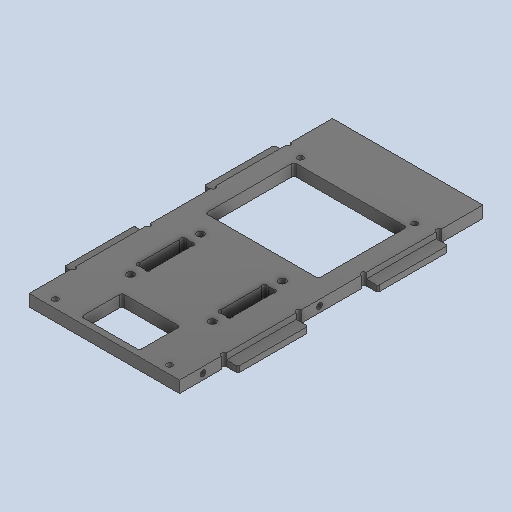
# Autodesk Inventor part: Cockpit_upper_bottom_frame
Saved by Autodesk Inventor 2022.4 (Build 264492000, 492)
## iProperties
Created: 2021-04-13
Part Number: Cockpit_upper_bottom_frame
Material: アセタール樹脂、黒
Document SubType Name: Modeling
Designer: Masato Kubotera
Density: 1.425 g/cm^3
Appearance: 滑らか - 黒
Mass: 43.5821 g
Surface Area: 172.155 cm^2
Volume: 30.5839 cm^3
Description: POM T5
d0: 64.500 mm
d1: 130.000 mm
d2: 20.000 mm
d3: 30.000 mm
d4: 30.000 mm
d5: 30.000 mm
d6: 1.050 mm
d7: 1.050 mm
d8: 1.050 mm
d9: 1.050 mm
d10: 5.000 mm
d23: 15.000 mm
d24: 5.000 mm
d25: 20.000 mm
d28: 3.100 mm
d66: 2.500 mm
d67: 0.00 deg
d68: 5.000 mm
d69: 0.00 deg
d72: 47.500 mm
d101: 1.000 mm
d103: 12.250 mm
d109: 71.250 mm
Author: Masato Kubotera
Title: Cockpit_horizontal_frame_02
Autodesk Inventor part; units mm, degrees
ref_plane "YZ Plane" through (0, 0, 0) normal (1, 0, 0) x (0, 1, 0)
ref_plane "XZ Plane" through (0, 0, 0) normal (0, 1, 0) x (-1, 0, 0)
ref_plane "XY Plane" through (0, 0, 0) normal (0, 0, 1) x (1, 0, 0)
sketch "スケッチ1" plane through (0, 0, 0) normal (0, 0, 1) x (1, 0, 0)
  line L0 (-32.25, 65) -> (32.25, 65)
  line L1 (32.25, 65) -> (32.25, 47.1)
  line L2 (-32.25, -65) -> (-32.25, -47.1)
  line L3 (-32.25, 65) -> (32.25, -65) construction
  line L4 (32.25, 65) -> (-32.25, -65) construction
  line L5 (-32.25, 45) -> (-37.25, 45)
  line L6 (-37.25, 15) -> (-32.25, 15)
  line L7 (-37.25, 15) -> (-37.25, 45)
  line L8 (-32.25, -15) -> (-37.25, -15)
  line L9 (-37.25, -15) -> (-37.25, -45)
  line L10 (-37.25, -45) -> (-32.25, -45)
  arc A0 (-32.25, 45) -> (-32.25, 47.1) centre (-32.25, 46.05) ccw
  arc A1 (-32.25, 12.9) -> (-32.25, 15) centre (-32.25, 13.95) ccw
  arc A2 (-32.25, -15) -> (-32.25, -12.9) centre (-32.25, -13.95) ccw
  arc A3 (-32.25, -47.1) -> (-32.25, -45) centre (-32.25, -46.05) ccw
  line L11 (-32.25, 47.1) -> (-32.25, 65)
  line L12 (-32.25, 12.9) -> (-32.25, 15) construction
  line L13 (-32.25, -12.9) -> (-32.25, 12.9)
  line L14 (-32.25, -47.1) -> (-32.25, -45) construction
  line L15 (0, 65) -> (0, -65) construction
  arc A4 (32.25, -45) -> (32.25, -47.1) centre (32.25, -46.05) ccw
  line L16 (37.25, -45) -> (32.25, -45)
  line L17 (37.25, -15) -> (37.25, -45)
  line L18 (32.25, -15) -> (37.25, -15)
  arc A5 (32.25, -12.9) -> (32.25, -15) centre (32.25, -13.95) ccw
  arc A6 (32.25, 15) -> (32.25, 12.9) centre (32.25, 13.95) ccw
  line L19 (37.25, 15) -> (37.25, 45)
  line L20 (37.25, 15) -> (32.25, 15)
  line L21 (32.25, 45) -> (37.25, 45)
  arc A7 (32.25, 47.1) -> (32.25, 45) centre (32.25, 46.05) ccw
  line L22 (32.25, 47.1) -> (32.25, 45) construction
  line L23 (32.25, 12.9) -> (32.25, -12.9)
  line L24 (32.25, -47.1) -> (32.25, -65)
  line L25 (32.25, -12.9) -> (32.25, -15) construction
  line L26 (-32.25, -15) -> (-32.25, -12.9) construction
  line L27 (-32.25, -45) -> (-32.25, -15)
  line L28 (32.25, -15) -> (32.25, -45)
  line L29 (32.25, -45) -> (32.25, -47.1) construction
  line L30 (-20, -11.25) -> (-15, -11.25) construction
  line L31 (-15, -11.25) -> (-15, -31.25) construction
  line L32 (-15, -31.25) -> (-20, -31.25) construction
  line L33 (-20, -31.25) -> (-20, -11.25) construction
  line L34 (-20, -11.25) -> (-15, -31.25) construction
  line L35 (-15, -11.25) -> (-20, -31.25) construction
  line L36 (-20, 2.5) -> (-15, 2.5) construction
  line L37 (-15, 2.5) -> (-15, -45) construction
  line L38 (-15, -45) -> (-20, -45) construction
  line L39 (-20, -45) -> (-20, 2.5) construction
  line L40 (-20, 2.5) -> (-15, -45) construction
  line L41 (-15, 2.5) -> (-20, -45) construction
  circle A8 centre (-17.5, -36.25) radius 1.55
  line L42 (-20, -21.25) -> (-15, -21.25) construction
  line L43 (-17.5, 2.5) -> (-17.5, -45) construction
  circle A9 centre (-17.5, -6.25) radius 1.55
  circle A10 centre (17.5, -36.25) radius 1.55
  circle A11 centre (17.5, -6.25) radius 1.55
  line L44 (32.25, -65) -> (16.75, -65)
  line L45 (-12.5, -62.5) -> (-12.5, -45)
  line L46 (-12.5, -45) -> (0, -45)
  line L47 (12.5, -62.5) -> (12.5, -45)
  line L48 (12.5, -45) -> (0, -45)
  line L49 (-16.75, -65) -> (-32.25, -65)
  line L50 (16.75, -65) -> (-16.75, -65)
  line L51 (-32.25, 45) -> (-32.25, 47.1) construction
  line L52 (-32.25, 15) -> (-32.25, 45)
  line L53 (32.25, 15) -> (32.25, 12.9) construction
  line L54 (32.25, 45) -> (32.25, 15)
  circle A12 centre (-24.5, 43.5) radius 1.25
  line L55 (-32.25, 0) -> (32.25, 0) construction
  line L56 (-32.25, 46.5) -> (32.25, 46.5) construction
  circle A13 centre (-24.5, -61.5) radius 1.25
  circle A14 centre (24.5, 43.5) radius 1.25
  circle A15 centre (24.5, -61.5) radius 1.25
  circle A16 centre (-17.5, -36.25) radius 3 construction
  line L57 (-12.5, -62.5) -> (12.5, -62.5)
  line L58 (-24.25, 40.5) -> (24.25, 40.5)
  line L59 (24.25, 2.5) -> (-24.25, 2.5)
  line L60 (-24.25, 2.5) -> (-24.25, 40.5)
  line L61 (24.25, 2.5) -> (24.25, 40.5)
  line L62 (-20.05, -29.8151) -> (-18.5651, -31.3) construction
  line L63 (-19.3075, -30.5575) -> (-20.05, -31.3) construction
  arc A17 (-20.05, -29.8151) -> (-18.5651, -31.3) centre (-19.3075, -30.5575) ccw
  line L64 (-20.05, -11.2) -> (-18.5651, -11.2) construction
  line L65 (-14.95, -11.2) -> (-14.95, -12.6849) construction
  line L66 (-14.95, -31.3) -> (-16.4349, -31.3) construction
  line L67 (-20.05, -31.3) -> (-20.05, -29.8151) construction
  line L68 (-20.05, -11.2) -> (-14.95, -31.3) construction
  line L69 (-14.95, -11.2) -> (-20.05, -31.3) construction
  arc A18 (-16.4349, -31.3) -> (-14.95, -29.8151) centre (-15.6925, -30.5575) ccw
  arc A19 (-18.5651, -11.2) -> (-20.05, -12.6849) centre (-19.3075, -11.9425) ccw
  arc A20 (-14.95, -12.6849) -> (-16.4349, -11.2) centre (-15.6925, -11.9425) ccw
  line L70 (-20.05, -29.8151) -> (-20.05, -12.6849)
  line L71 (-18.5651, -31.3) -> (-20.05, -31.3) construction
  line L72 (-16.4349, -31.3) -> (-18.5651, -31.3)
  line L73 (-14.95, -29.8151) -> (-14.95, -31.3) construction
  line L74 (-20.05, -12.6849) -> (-20.05, -11.2) construction
  line L75 (-18.5651, -11.2) -> (-16.4349, -11.2)
  line L76 (-16.4349, -11.2) -> (-14.95, -11.2) construction
  line L77 (-14.95, -12.6849) -> (-14.95, -29.8151)
  arc A21 (18.5651, -31.3) -> (20.05, -29.8151) centre (19.3075, -30.5575) ccw
  arc A22 (14.95, -29.8151) -> (16.4349, -31.3) centre (15.6925, -30.5575) ccw
  arc A23 (16.4349, -11.2) -> (14.95, -12.6849) centre (15.6925, -11.9425) ccw
  arc A24 (20.05, -12.6849) -> (18.5651, -11.2) centre (19.3075, -11.9425) ccw
  line L78 (20.05, -29.8151) -> (20.05, -12.6849)
  line L79 (16.4349, -31.3) -> (18.5651, -31.3)
  line L80 (18.5651, -11.2) -> (16.4349, -11.2)
  line L81 (14.95, -12.6849) -> (14.95, -29.8151)
  line L82 (-32.25, -65) -> (-32.25, -70)
  line L83 (-32.25, -70) -> (32.25, -70)
  line L84 (32.25, -70) -> (32.25, -65)
  point P0 (0, 0)
  point P1 (0, 0)
  point P2 (0, 0)
  point P3 (28, 15)
  point P4 (28, 45)
  point P5 (-17.5, -21.25)
  point P6 (28, 45)
  point P7 (28, 15)
  dimension "d0" = 64.5
  dimension "d1" = 130
  dimension "d2" = 20
  dimension "d3" = 30
  dimension "d4" = 30
  dimension "d5" = 30
  dimension "d6" = 1.05
  dimension "d7" = 1.05
  dimension "d8" = 1.05
  dimension "d9" = 1.05
  dimension "d10" = 5
  dimension "d23" = 15
  dimension "d24" = 5
  dimension "d25" = 20
  dimension "d28" = 3.1
  dimension "d72" = 47.5
  dimension "d103" = 12.25
  dimension "d109" = 71.25
  dimension "d111" = 20
  dimension "d113" = 7.75
  dimension "d114" = 2.5
  dimension "d115" = 18.5
  dimension "d116" = 3
  dimension "d117" = 2.5
  dimension "d118" = 7.75
  dimension "d119" = 3.5
  dimension "d120" = 25
  dimension "d121" = 6
  dimension "d124" = 2.5
  dimension "d126" = 8
  dimension "d128" = 6
  dimension "d130" = 1.05
  dimension "d131" = 0.05
  dimension "d132" = 0.05
  dimension "d133" = 5
  dimension "d157" = 25
  dimension "d158" = 30
  constraints: 168 end point, 95 parallel, 52 perpendicular, 46 symmetric about line, 40 point on circle, 25 centre point, 22 midpoint, 15 horizontal, 10 vertical, 6 point on line, 3 coincident, 3 collinear, 30 other
  measures "d0" distance of L0.start L0.end
  measures "d1" distance of L0.end L3.end
  measures "d2" distance between parallel lines of L5 L0
  measures "d3" distance of L6.start L5.end
  measures "d4" distance between parallel lines of L8 L6
  measures "d5" distance of L8.end L9.end
  measures "d6" radius of A0
  measures "d7" radius of A1
  measures "d8" radius of A2
  measures "d9" radius of A3
  measures "d10" distance between parallel lines of L7 L11
  measures "d23" distance between parallel lines of L15 L31
  measures "d24" distance of L31.end L32.end
  measures "d25" distance of L30.end L31.end
  measures "d28" diameter of A8
  measures "d72" distance of L36.end L37.end
  measures "d109" distance from line of L0 A9.centre
  measures "d111" distance between parallel lines of L44 L46
  measures "d113" distance from line of A12.centre L11
  measures "d114" diameter of A12
  measures "d115" distance between parallel lines of L56 L0
  measures "d116" distance from line of L56 A12.centre
  measures "d117" diameter of A13
  measures "d119" distance from line of L49 A13.centre
  measures "d120" distance between parallel lines of L47 L45
  measures "d121" diameter of A16
  measures "d124" distance between parallel lines of L50 L57
  measures "d126" distance between parallel lines of L60 L52
  measures "d128" distance between parallel lines of L58 L56
  measures "d130" radius of A17
  measures "d131" distance between parallel lines of L72 L32
  measures "d132" distance between parallel lines of L70 L39
  measures "d133" distance of L4.end L82.end
  measures "d157" distance between parallel lines of L83 L38
  measures "d158" distance of A8.centre A9.centre
extrude "押し出し1" add sketch "スケッチ1" along normal blind 2.5 contours L0 L1 A7 L54 A6 L23 A5 L28 A4 L24 L44 L50 L49 L2 A3 L27 A2 L13 A1 L52 A0 L11 | L52 L6 L7 L5 | L21 L19 L20 L54 | L27 L10 L9 L8 | L18 L17 L16 L28
extrude "押し出し2" add sketch "スケッチ1" along normal blind 5 contours L0 L1 A7 L54 A6 L23 A5 L28 A4 L24 L44 L50 L49 L2 A3 L27 A2 L13 A1 L52 A0 L11
fillet "フィレット1" radius 1 7 edges at (-12.5, -45, 2.5) (-12.5, -62.5, 2.5) (12.5, -62.5, 2.5) (-24.25, 40.5, 2.5) (24.25, 40.5, 2.5) (24.25, 2.5, 2.5) (-24.25, 2.5, 2.5)
sketch "スケッチ7" plane through (32.25, -70, 0) normal (1, 0, 0) x (0, 0, -1)
  line L0 (0, 55) -> (-2.5, 55) projected
  line L1 (0, 57.1) -> (0, 82.9) projected
  line L2 (0, 5) -> (0, 22.9) projected
  point P0 (0, 70)
  point P1 (-2.5, 15)
  point P2 (-2.5, 65)
  point P3 (0, 25)
  dimension "d136" = 10
  dimension "d137" = 10
  dimension "d138" = 2.5
  dimension "d139" = 2.5
  measures "d136" vertical distance of point (0, 25) point (-2.5, 15)
  measures "d137" distance from line of point (-2.5, 65) L0
  measures "d138" distance from line of L1 point (-2.5, 65)
  measures "d139" distance from line of L2 point (-2.5, 15)
hole "穴6" at (32.25, -55, 2.5) at (32.25, -5, 2.5) direction (-1, 0, 0) diameter 2.459 depth 4 thread size "M3x0.5" class "6H" standard "ISO Metric profile"
sketch "スケッチ8" plane through (-32.25, -70, 0) normal (-1, 0, 0) x (0, 0, 1)
  circle A0 centre (2.5, 15) radius 1.2295 projected
  circle A1 centre (2.5, 65) radius 1.2295 projected
  point P0 (0, 70)
  point P1 (2.5, 15)
  point P2 (2.5, 65)
  constraints: 2 coincident
hole "穴7" at (-32.25, -5, 2.5) at (-32.25, -55, 2.5) direction (1, 0, 0) diameter 2.459 depth 4 thread size "M3x0.5" class "6H" standard "ISO Metric profile"
chamfer "面取り2" distance 0.5 angle 45 8 edges at (-37.25, -45, 1.25) (-37.25, -15, 1.25) (-37.25, 15, 1.25) (-37.25, 45, 1.25) (37.25, 15, 1.25) (37.25, 45, 1.25) (37.25, -15, 1.25) (37.25, -45, 1.25)
equation "\"d2\" = -0.5 * d4 + 0.5 * d1 - d3"
equation "\"d5\" = d3"
equation "\"d7\" = d6"
equation "\"d8\" = d7"
equation "\"d9\" = d8"
